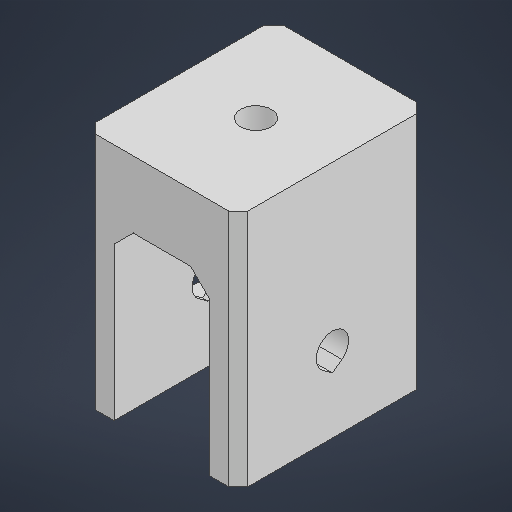
# Autodesk Inventor part: Idlert Tensioner
Saved by Autodesk Inventor 2025.1 (Build 291241000, 241)
## iProperties
Created: 2025-01-23
Part Number: Idlert Tensioner
Material: Generic
Document SubType Name: Modeling
Designer: jerem
Density: 1 g/cm^3
Appearance: Default
Author: jerem
## iProperties of the stored document Idlert Tensioner_3DPrint.ipt
Created: 2025-01-23
Part Number: Idlert Tensioner_3DPrint
Material: Generic
Document SubType Name: Modeling
Designer: jerem
Density: 1 g/cm^3
Appearance: Default
Author: jerem
Autodesk Inventor part; units mm, degrees
ref_plane "YZ Plane" through (0, 0, 0) normal (1, 0, 0) x (0, 1, 0)
ref_plane "XZ Plane" through (0, 0, 0) normal (0, 1, 0) x (-1, 0, 0)
ref_plane "XY Plane" through (0, 0, 0) normal (0, 0, 1) x (1, 0, 0)
sketch "Sketch3" plane through (0, 0, 0) normal (0, 1, 0) x (-1, 0, 0)
  line L0 (-8, 9.85) -> (8, 9.85)
  line L1 (8, 9.85) -> (8, -9.85)
  line L2 (8, -9.85) -> (-8, -9.85)
  line L3 (-8, -9.85) -> (-8, 9.85)
  line L4 (-8, 9.85) -> (8, -9.85) construction
  line L5 (8, 9.85) -> (-8, -9.85) construction
  line L6 (5, -9.85) -> (5, 9.85)
  line L7 (-5, 9.85) -> (-5, -9.85)
  line L8 (-5, -6.1562) -> (5, -6.1562) construction
  point P0 (0, 0)
  dimension "d12" = 19.7
  dimension "d36" = 10
  dimension "d52" = 16
  constraints: 18 end point, 8 point on line, 3 perpendicular, 2 horizontal, 2 midpoint, 2 parallel
  measures "d12" distance of L0.end L1.end
  measures "d36" distance between parallel lines of L7 L6
  measures "d52" distance of L0.end L0.start
extrude "Extrusion3" add sketch "Sketch3" along normal blind 25
sketch "Sketch4" plane through (8, 0, 9.85) normal (1, 0, 0) x (0, 0, -1)
  line L0 (9.85, 0) -> (9.85, 8) construction
  circle A0 centre (9.85, 8) radius 1.7
  line L1 (0, 0) -> (19.7, 0) projected
  line L2 (9.85, 5.9) -> (10.848, 6.6238)
  line L3 (8.852, 6.6238) -> (9.85, 5.9)
  dimension "d15" = 3.4
  dimension "d16" = 8
  dimension "d53" = 2.1
  constraints: 6 end point, 2 point on circle, 2 tangent, 1 centre point, 1 coincident, 1 point on line, 1 vertical
  measures "d15" diameter of A0
  measures "d16" distance from line of L1 L0.end
  measures "d53" distance of L0.end L2.start
extrude "Extrusion4" cut sketch "Sketch3" along normal blind 18 contours L0 L6 L2 L7
extrude "Extrusion5" cut sketch "Sketch4" against normal through all
sketch "Sketch7" plane through (0, 25, 0) normal (0, 1, 0) x (1, 0, 0)
  circle A0 centre (0, 0) radius 1.6
  circle A1 centre (0, 0) radius 3.6
  line L0 (-5, 10) -> (5, -10) construction
  line L1 (8, 9.85) -> (-8, 9.85) projected
  line L2 (-8, 9.85) -> (-8, -9.85) projected
  line L3 (-8, -9.85) -> (8, -9.85) projected
  line L4 (8, -9.85) -> (8, 9.85) projected
  line L5 (-8, 9.85) -> (8, -9.85) construction
  line L6 (8, 9.85) -> (-8, -9.85) construction
  dimension "d30" = 3.2
  dimension "d47" = 7.2
  constraints: 4 end point, 2 centre point, 1 coincident, 1 midpoint
  measures "d30" diameter of A0
  measures "d47" diameter of A1
extrude "Extrusion8" cut sketch "Sketch7" along normal through all both and the other way through all contours A0
extrude "Extrusion9" cut sketch "Sketch7" along normal blind 3 from surface at -7 contours A1
chamfer "Chamfer2" distance 2 angle 45 2 edges at (5, 18, 0) (-5, 18, 0)
chamfer "Chamfer3" distance 1 angle 45 4 edges at (-8, 12.5, 9.85) (-8, 12.5, -9.85) (8, 12.5, -9.85) (8, 12.5, 9.85)
sketch "Sketch9" plane through (-8, 0, -8.85) normal (-1, 0, 0) x (0, 0, 1)
  arc A0 (9.848, 6.6238) -> (7.852, 6.6238) centre (8.85, 8) ccw projected
  line L0 (6.05, 5.15) -> (11.65, 5.15)
  line L1 (11.65, 5.15) -> (11.65, 10.85)
  line L2 (11.65, 10.85) -> (6.05, 10.85)
  line L3 (6.05, 10.85) -> (6.05, 5.15)
  line L4 (6.05, 5.15) -> (11.65, 10.85) construction
  line L5 (11.65, 5.15) -> (6.05, 10.85) construction
  point P0 (8.85, 0)
  dimension "d57" = 5.6
  dimension "d58" = 5.7
  constraints: 12 end point, 2 midpoint, 2 parallel, 1 horizontal, 1 perpendicular
  measures "d57" distance of L2.end L1.end
  measures "d58" distance of L1.end L0.end
extrude "Extrusion10" cut sketch "Sketch9" against normal blind 2.4
body "Solid2"
